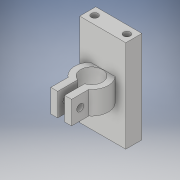
# Autodesk Inventor part: zaxis_clamp1
Saved by Autodesk Inventor 2019 (Build 230136000, 136)
## iProperties
Created: 2020-02-02
Material: Generic
Document SubType Name: Modeling
Designer: Nishant
Density: 1 g/cm^3
Appearance: Default
Author: Nishant
Autodesk Inventor part; units mm, degrees
ref_plane "YZ Plane" through (0, 0, 0) normal (1, 0, 0) x (0, 1, 0)
ref_plane "XZ Plane" through (0, 0, 0) normal (0, 1, 0) x (-1, 0, 0)
ref_plane "XY Plane" through (0, 0, 0) normal (0, 0, 1) x (1, 0, 0)
sketch "Sketch1" plane through (0, 0, 0) normal (0, 1, 0) x (-1, 0, 0)
  arc A0 (-1.5, 9.2569) -> (1.5, 9.2569) centre (0, 4.75) ccw
  arc A1 (5.3889, -0.1) -> (4.5, 10.4344) centre (0, 4.75) ccw
  arc A2 (-4.5, 10.4344) -> (-5.3889, -0.1) centre (0, 4.75) ccw
  line L0 (-4.5, 10.4344) -> (-4.5, 17.9344)
  line L1 (4.5, 10.4344) -> (4.5, 17.9344)
  line L2 (-1.5, 9.2569) -> (-1.5, 17.9344)
  line L3 (1.5, 9.2569) -> (1.5, 17.9344)
  line L4 (4.5, 17.9344) -> (1.5, 17.9344)
  line L5 (-1.5, 17.9344) -> (-4.5, 17.9344)
  line L6 (5.3889, -0.1) -> (-5.3889, -0.1)
  point P0 (0, 0)
  constraints: 14 end point, 6 point on circle, 4 perpendicular, 3 centre point, 3 horizontal, 2 vertical, 1 coincident
extrude "Extrusion1" add sketch "Sketch1" along normal blind 10
sketch "Sketch2" plane through (0, 0, 0) normal (0, 1, 0) x (-1, 0, 0)
  line L0 (-5.3889, -0.1) -> (5.3889, -0.1) projected
  line L1 (0, -0.1) -> (-10, -0.1)
  line L2 (0, -0.1) -> (10, -0.1)
  line L3 (-10, -0.1) -> (-10, -7.1)
  line L4 (-10, -7.1) -> (10, -7.1)
  line L5 (10, -7.1) -> (10, -0.1)
  point P0 (0, 0)
  dimension "d13" = 10
  dimension "d14" = 10
  dimension "d15" = 7
  dimension "d16" = 20
  dimension "d17" = 7
  constraints: 10 end point, 1 collinear, 1 midpoint, 1 perpendicular, 1 point on line, 1 vertical
  measures "d13" distance of L1.start L1.end
  measures "d14" distance of L1.start L2.end
  measures "d15" distance of L1.end L3.end
  measures "d16" distance of L3.end L4.end
  measures "d17" distance of L4.end L2.end
extrude "Extrusion2" add sketch "Sketch2" along normal blind 25 and the other way blind 15
sketch "Sketch3" plane through (0, 25, 0) normal (0, 1, 0) x (1, 0, 0)
  line L0 (-10, 0.1) -> (10, 0.1) projected
  line L1 (10, 7.1) -> (10, 0.1) projected
  circle A0 centre (7, 3.6) radius 1.5
  line L2 (-10, 7.1) -> (-10, 0.1) projected
  circle A1 centre (-7, 3.6) radius 1.5
  point P0 (0, 0)
  dimension "d24" = 3
  dimension "d27" = 3
  constraints: 2 centre point
  measures "d24" diameter of A0
  measures "d27" diameter of A1
hole "Hole1" at (-7, 25, -3.6) at (7, 25, -3.6) direction (0, -1, 0) diameter 3 end through all both
sketch "Sketch4" plane through (4.5, 0, 17.9344) normal (1, 0, 0) x (0, 0, -1)
  line L0 (0, 10) -> (8.6775, 10) projected
  circle A0 centre (3.75, 5) radius 1.5
  point P0 (17.9344, 0)
  point P1 (0, 0)
  point P2 (7.5, 0)
  dimension "d36" = 3
  constraints: 1 centre point
  measures "d36" diameter of A0
hole "Hole2" at (4.5, 5, 14.1844) direction (-1, 0, 0) diameter 3 end through all both
body "Solid1"
